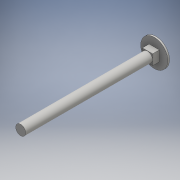
# Autodesk Inventor part: wagon_bolt
Saved by Autodesk Inventor 2016 (Build 200138000, 138)
## iProperties
Created: 2017-01-01
Part Number: wagon_bolt
Material: Generic
Document SubType Name: Modeling
Designer: hesaon
Density: 1 g/cm^3
Appearance: Default
Author: hesaon
Autodesk Inventor part; units mm, degrees
ref_plane "YZ Plane" through (0, 0, 0) normal (1, 0, 0) x (0, 1, 0)
ref_plane "XZ Plane" through (0, 0, 0) normal (0, 1, 0) x (-1, 0, 0)
ref_plane "XY Plane" through (0, 0, 0) normal (0, 0, 1) x (1, 0, 0)
sketch "Sketch4" plane through (0, 0, 0) normal (0, 0, 1) x (1, 0, 0)
  line L0 (0, 0) -> (0, 3)
  line L1 (0, 0) -> (8.05, 0)
  line L2 (8.05, 0) -> (8.05, 1)
  arc A0 (8.05, 1) -> (0, 3) centre (0.2076, -13.3651) ccw
  dimension "d7" = 3
  dimension "d8" = 8.05
  dimension "d9" = 1
  constraints: 6 end point, 2 point on circle, 1 centre point, 1 horizontal, 1 perpendicular, 1 vertical
  measures "d7" distance of L0.start L0.end
  measures "d8" distance of L0.start L1.end
  measures "d9" distance of L1.end L2.end
revolve "Revolution1" add sketch "Sketch4" angle 360 about axis through (0, 0, 0) along (0, 1, 0)
sketch "Sketch5" plane through (0, 0, 0) normal (0, -1, 0) x (1, 0, 0)
  line L0 (3.05, 3.05) -> (-3.05, 3.05)
  line L1 (-3.05, 3.05) -> (-3.05, -3.05)
  line L2 (-3.05, -3.05) -> (3.05, -3.05)
  line L3 (3.05, -3.05) -> (3.05, 3.05)
  point P0 (0, 0)
  dimension "d11" = 6.1
  dimension "d12" = 6.1
  dimension "d13" = 3.05
  dimension "d14" = 3.05
  constraints: 8 end point, 2 parallel, 1 horizontal, 1 perpendicular
  measures "d11" distance of L2.end L1.end
  measures "d12" distance of L1.end L0.end
  measures "d13" distance from line of L3 point (0, 0)
  measures "d14" distance from line of point (0, 0) L0
extrude "Extrusion2" add sketch "Sketch5" along normal blind 4
sketch "Sketch6" plane through (0, -4, 0) normal (0, -1, 0) x (1, 0, 0)
  circle A0 centre (0, 0) radius 2.945
  dimension "d17" = 5.89
  constraints: 1 centre point, 1 coincident
  measures "d17" diameter of A0
extrude "Extrusion3" add sketch "Sketch6" along normal blind 75.5
body "Solid2"
